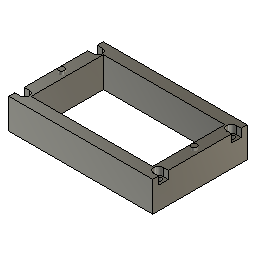
Flip Jig v5 (Autodesk Fusion 360 design; units mm, degrees)
Autodesk Fusion 360 part; units mm, degrees
sketch "Sketch1" plane through (0, 0, 0) normal (0, 0, 1) x (1, 0, 0)
  line L0 (11.0732, 10.0806) -> (161.9332, 10.0806)
  line L1 (161.9332, 10.0806) -> (161.9332, 109.0806)
  line L2 (161.9332, 109.0806) -> (11.0732, 109.0806)
  line L3 (11.0732, 109.0806) -> (11.0732, 10.0806)
  line L4 (22.8832, 21.7056) -> (150.1332, 21.7056)
  line L5 (150.1332, 21.7056) -> (150.1332, 97.4556)
  line L6 (150.1332, 97.4556) -> (22.8832, 97.4556)
  line L7 (22.8832, 97.4556) -> (22.8832, 21.7056)
  dimension "d1" = 150.86
  dimension "d2" = 99
  dimension "d3" = 127.25
  dimension "d4" = 75.75
  dimension "d5" = 11.625
  dimension "d6" = 11.8
  constraint horizontal L0
  constraint vertical L1
  constraint horizontal L2
  constraint vertical L3
  constraint horizontal L4
  constraint vertical L5
  constraint horizontal L6
  constraint vertical L7
  measures "d1" distance of L0.start L0.end
  measures "d2" distance of L0.start L2.end
  measures "d3" distance of L4.start L4.end
  measures "d4" distance of L4.start L6.end
  measures "d5" distance of L2 L6
  measures "d6" distance of L1 L5
extrude "Extrude1" add sketch "Sketch1" along normal blind 31.66 makes body 1
sketch "Sketch2" plane through (0, 0, 31.66) normal (0, 0, 1) x (-1, 0, 0)
  line L0 (-22.8832, -21.7056) -> (-22.8832, -97.4556)
  line L1 (-22.8832, -97.4556) -> (-150.1332, -97.4556)
  line L2 (-150.1332, -97.4556) -> (-150.1332, -21.7056)
  line L3 (-150.1332, -21.7056) -> (-22.8832, -21.7056)
  line L4 (-11.0732, -109.0806) -> (-11.0732, -10.0806)
  line L5 (-11.0732, -10.0806) -> (-161.9332, -10.0806)
  line L6 (-161.9332, -10.0806) -> (-161.9332, -109.0806)
  line L7 (-161.9332, -109.0806) -> (-11.0732, -109.0806)
  line L8 (-11.0732, -10.0806) -> (-11.0732, -16.3306) construction
  line L9 (-11.0732, -109.0806) -> (-11.0732, -102.8306) construction
  line L10 (-161.9332, -109.0806) -> (-161.9332, -102.8306) construction
  line L11 (-161.9332, -10.0806) -> (-161.9332, -16.3306) construction
  circle A0 centre (-156.6332, -21.3306) radius 5
  line L12 (-161.9332, -16.3306) -> (-156.6512, -16.3306)
  line L13 (-156.665, -26.3305) -> (-161.9332, -26.3305)
  line L14 (-156.665, -26.3305) -> (-161.9332, -26.3305)
  line L15 (-161.9332, -26.3305) -> (-161.9332, -16.3306)
  line L16 (-161.9332, -16.3306) -> (-156.665, -16.3306)
  line L17 (-156.665, -16.3306) -> (-156.665, -26.3305)
  circle A1 centre (-156.6332, -97.831) radius 5
  line L18 (-156.6951, -92.8306) -> (-156.6951, -102.8306)
  line L19 (-156.6951, -102.8306) -> (-161.9396, -102.8306)
  line L20 (-161.9396, -102.8306) -> (-161.9396, -92.8306)
  line L21 (-161.9396, -92.8306) -> (-156.6951, -92.8306)
  line L22 (-156.6951, -92.8306) -> (-156.6951, -102.8306)
  circle A2 centre (-16.3832, -97.8306) radius 5
  line L23 (-11.0732, -102.8306) -> (-16.6232, -102.8306)
  line L24 (-16.6232, -102.8306) -> (-16.6232, -92.8306)
  line L25 (-16.6232, -92.8306) -> (-11.0732, -92.8306)
  line L26 (-11.0732, -92.8306) -> (-11.0732, -102.8306)
  circle A3 centre (-16.3832, -21.3306) radius 5
  line L27 (-11.0732, -16.3306) -> (-16.4732, -16.3306)
  line L28 (-16.4732, -16.3306) -> (-16.4732, -26.3306)
  line L29 (-16.4732, -26.3306) -> (-11.0732, -26.3306)
  line L30 (-11.0732, -26.3306) -> (-11.0732, -16.3306)
  dimension "d9" = 6.25
  dimension "d10" = 6.25
  dimension "d11" = 6.25
  dimension "d12" = 6.25
  dimension "d13" = 10
  dimension "d14" = 6.5
  dimension "d15" = 5
  dimension "d20" = 10
  dimension "d23" = 6.5
  dimension "d24" = 10
  dimension "d29" = 6.25
  dimension "d30" = 10
  dimension "d33" = 10
  dimension "d34" = 11.25
  dimension "d35" = 6.5
  dimension "d36" = 5.55
  dimension "d37" = 10
  dimension "d40" = 10
  dimension "d41" = 11.25
  dimension "d42" = 6.5
  dimension "d43" = 10
  dimension "d44" = 5.4
  constraint coincident L4.end L5.start
  constraint perpendicular L5 L8
  constraint coincident L4.start L7.end
  constraint perpendicular L7 L9
  constraint coincident L6.end L7.start
  constraint perpendicular L7 L10
  constraint coincident L5.end L6.start
  constraint perpendicular L5 L11
  constraint horizontal L12
  constraint horizontal L13
  constraint coincident A0 L13.start
  constraint coincident L6 L13.end
  constraint horizontal L14
  constraint vertical L15
  constraint horizontal L16
  constraint vertical L17
  constraint vertical L18
  constraint coincident A1 L18.end
  constraint horizontal L19
  constraint vertical L20
  constraint horizontal L21
  constraint vertical L22
  constraint horizontal L23
  constraint vertical L24
  constraint horizontal L25
  constraint vertical L26
  constraint horizontal L27
  constraint vertical L28
  constraint horizontal L29
  constraint vertical L30
  measures "d9" distance of L4.end L8.end
  measures "d10" distance of L4.start L9.end
  measures "d11" distance of L6.end L10.end
  measures "d12" distance of L5.end L11.end
  measures "d13" diameter of A0
  measures "d14" distance of L2 A0.centre
  measures "d15" distance of A0.centre L12
  measures "d20" diameter of A1
  measures "d23" distance of L2 A1.centre
  measures "d24" distance of L18.end L18.start
  measures "d29" distance of L7 L18.end
  measures "d30" distance of L18.end L18.start
  measures "d33" diameter of A2
  measures "d34" distance of L7 A2.centre
  measures "d35" distance of L0 A2.centre
  measures "d36" distance of L9.end L23.end
  measures "d37" distance of L9.end L25.end
  measures "d40" diameter of A3
  measures "d41" vertical distance of L4.end A3.centre
  measures "d42" distance of L0 A3.centre
  measures "d43" distance of L8.end L29.end
  measures "d44" distance of L8.end L27.end
extrude "Extrude6" cut sketch "Sketch2" against normal blind 8.3 contours L4 A2 L23 L25 L26 | A2 L24 | A2 L24 bodies 1
extrude "Extrude5" cut sketch "Sketch2" against normal blind 8.3 contours L6 A1 L19 L21 | A1 L18 L22 | A1 L18 L22 bodies 1
extrude "Extrude4" cut sketch "Sketch2" against normal blind 8.3 contours L6 A1 L19 L21 | A1 L18 L22 | A1 L18 L22 bodies 1
extrude "Extrude2" cut sketch "Sketch2" against normal blind 8.3 contours A0 L12 L17 | A0 L17 bodies 1
extrude "Extrude3" cut sketch "Sketch2" against normal blind 8.3 contours L6 A0 L12 L13 L14 L15 L16 bodies 1
extrude "Extrude7" cut sketch "Sketch2" against normal blind 8.3 contours L4 A3 L27 L29 L30 | A3 L28 | A3 L28 bodies 1
sketch "Sketch3" plane through (0, 0, 31.66) normal (0, 0, 1) x (-1, 0, 0)
  line L0 (-11.0732, -26.3306) -> (-16.3832, -26.3306)
  arc A0 (-16.3832, -16.3306) -> (-16.3832, -26.3306) centre (-16.3832, -21.3306) ccw
  line L1 (-16.3832, -16.3306) -> (-11.0732, -16.3306)
  line L2 (-11.0732, -16.3306) -> (-11.0732, -10.0806)
  line L3 (-11.0732, -10.0806) -> (-161.9332, -10.0806)
  line L4 (-161.9332, -10.0806) -> (-161.9332, -16.3306)
  line L5 (-161.9332, -16.3306) -> (-156.665, -16.3306)
  line L6 (-156.665, -16.3306) -> (-156.665, -16.3307)
  arc A1 (-156.665, -26.3305) -> (-156.665, -16.3307) centre (-156.6332, -21.3306) ccw
  line L7 (-156.665, -26.3305) -> (-161.9332, -26.3305)
  line L8 (-161.9332, -26.3305) -> (-161.9332, -92.8306)
  line L9 (-161.9332, -92.8306) -> (-156.6951, -92.8306)
  line L10 (-156.6951, -92.8306) -> (-156.6951, -92.8314)
  arc A2 (-156.6951, -102.8306) -> (-156.6951, -92.8314) centre (-156.6332, -97.831) ccw
  line L11 (-156.6951, -102.8306) -> (-161.9332, -102.8306)
  line L12 (-161.9332, -102.8306) -> (-161.9332, -109.0806)
  line L13 (-161.9332, -109.0806) -> (-11.0732, -109.0806)
  line L14 (-11.0732, -109.0806) -> (-11.0732, -102.8306)
  line L15 (-11.0732, -102.8306) -> (-16.3832, -102.8306)
  arc A3 (-16.3832, -92.8306) -> (-16.3832, -102.8306) centre (-16.3832, -97.8306) ccw
  line L16 (-16.3832, -92.8306) -> (-11.0732, -92.8306)
  line L17 (-11.0732, -92.8306) -> (-11.0732, -26.3306)
  line L18 (-22.8832, -21.7056) -> (-22.8832, -97.4556)
  line L19 (-22.8832, -97.4556) -> (-150.1332, -97.4556)
  line L20 (-150.1332, -97.4556) -> (-150.1332, -21.7056)
  line L21 (-150.1332, -21.7056) -> (-22.8832, -21.7056)
  circle A4 centre (-16.3832, -97.8306) radius 3
  circle A5 centre (-16.3832, -21.3306) radius 3
  circle A6 centre (-156.6332, -97.831) radius 3
  circle A7 centre (-156.6332, -21.3306) radius 3
  dimension "d48" = 6
  dimension "d49" = 6
  dimension "d50" = 6
  dimension "d51" = 6
  constraint concentric A3 A4
  constraint concentric A0 A5
  constraint concentric A2 A6
  constraint concentric A1 A7
  measures "d48" diameter of A4
  measures "d49" diameter of A5
  measures "d50" diameter of A6
  measures "d51" diameter of A7
extrude "Extrude8" cut sketch "Sketch3" against normal up to surface (31.66 mm away) contours A4 | A5 | A6 | A7 bodies 1
sketch "Sketch4" plane through (0, 0, 0) normal (0, 0, 1) x (1, 0, 0)
  line L0 (161.9332, 109.0806) -> (11.0732, 109.0806) construction
  line L1 (150.1332, 97.4556) -> (150.1332, 21.7056) construction
  line L2 (150.1332, 59.5806) -> (156.0332, 59.5806) construction
  circle A0 centre (156.0332, 59.5806) radius 2.95
  line L3 (22.8832, 21.7056) -> (22.8832, 97.4556) construction
  line L4 (11.0732, 92.8306) -> (11.0732, 26.3306) construction
  circle A1 centre (16.9782, 59.5806) radius 2.95
  point P0 (156.6951, 92.8314)
  dimension "d55" = 5.9
  dimension "d56" = 5.9
  dimension "d59" = 5.9
  constraint midpoint L1 L2.start
  constraint coincident L2.end A0.centre
  measures "d55" distance of L2.start L2.end
  measures "d56" diameter of A0
  measures "d59" diameter of A1
sketch "Sketch5" plane through (0, 0, 0) normal (0, 0, 1) x (1, 0, 0)
  circle A0 centre (16.9782, 59.5806) radius 2.95
  circle A1 centre (156.0332, 59.5806) radius 2.95
  point P0 (16.9782, 59.5806)
  point P1 (156.0332, 59.5806)
  dimension "d60" = 5.9
  dimension "d61" = 5.9
  constraint coincident P0 A0.centre
  constraint coincident P1 A1.centre
  measures "d60" diameter of A0
  measures "d61" diameter of A1
extrude "Extrude9" add sketch "Sketch4" along normal blind 34.66 separate body makes body 2 at (156.8322, 62.4203, 23.1067) makes body 3 at (19.9245, 59.4336, 23.1067)
extrude "Extrude10" add 2 faces at (15.285, 58.7652, 0) (155.6739, 57.5574, 0) along direction (0, 0, -1) blind 3 separate body on bodies 2 3 makes body 4 at (19.9245, 59.4336, -2) makes body 5 at (156.8322, 62.4203, -2)
equation "d5 = ( ( 99 - 75.75 ) / 2 ) * 1 mm"
equation "d6 = ( ( 150.85 - 127.25 ) / 2 ) * 1 mm"
equation "d7 = bodyH"
equation "d34 = 6.25 mm + 5 mm"
equation "d41 = 6.25 mm + 5 mm"
equation "d55 = ( 11.800 / 2 ) * 1 mm"
equation "d62 = bodyH + 3 mm"
equation "bodyH = 31.66 mm" comment "31.66 for Nomad 883 Pro"
